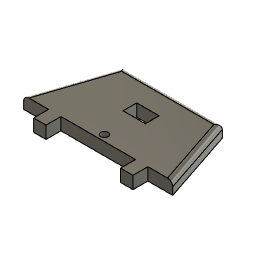
supporti_termice_1.2 (Autodesk Fusion 360 design; units mm, degrees)
Autodesk Fusion 360 part; units mm, degrees
sketch "Sketch1" plane through (0, 0, 0) normal (0, 1, 0) x (1, 0, 0)
  line L0 (-15, 0) -> (-15, -6)
  line L1 (-15, -6) -> (-20, -6)
  line L2 (-20, -6) -> (-20, 0)
  line L3 (15, 0) -> (15, -6)
  line L4 (15, -6) -> (20, -6)
  line L5 (20, -6) -> (20, 0)
  line L6 (-15, 0) -> (15, 0)
  line L7 (20, 0) -> (30, 0)
  line L8 (-20, 0) -> (-30, 0)
  line L9 (-30, 0) -> (-20, 30)
  line L10 (-20, 30) -> (0, 30)
  line L11 (0, 30) -> (20, 30)
  line L12 (20, 30) -> (30, 0)
  line L13 (0, 20) -> (-4.5, 20)
  line L14 (-4.5, 20) -> (-4.5, 14.5)
  line L15 (-4.5, 14.5) -> (4.5, 14.5)
  line L16 (0, 20) -> (4.5, 20)
  line L17 (4.5, 20) -> (4.5, 14.5)
  circle A0 centre (0, 2.5) radius 1.5
  dimension "d15" = 3
  constraint perpendicular L0 L1
  constraint perpendicular L1 L2
  constraint perpendicular L3 L6
  constraint perpendicular L5 L7
  constraint perpendicular L2 L8
  constraint perpendicular L2 L10
  constraint parallel L10 L11
  constraint horizontal L13
  constraint perpendicular L13 L14
  constraint perpendicular L14 L15
  constraint parallel L13 L16
  measures "d15" diameter of A0
extrude "Extrude2" add sketch "Sketch1" along normal blind 5
fillet "Fillet2" radius 2 3 edges at (0, 5, -30) (-25, 5, -15) (25, 5, -15)
